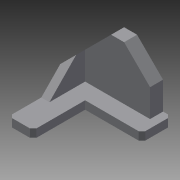
# Autodesk Inventor part: z-axis-bottom
Saved by Autodesk Inventor 2015 (Build 190159000, 159)
## iProperties
Created: 2015-05-29
Part Number: z-axis-bottom
Material: Generic
Document SubType Name: Modeling
Designer: X
Density: 1 g/cm^3
Appearance: Default
Author: X
Autodesk Inventor part; units mm, degrees
ref_plane "YZ Plane" through (0, 0, 0) normal (1, 0, 0) x (0, 1, 0)
ref_plane "XZ Plane" through (0, 0, 0) normal (0, 1, 0) x (-1, 0, 0)
ref_plane "XY Plane" through (0, 0, 0) normal (0, 0, 1) x (1, 0, 0)
sketch "Sketch2" plane through (0, 0, 0) normal (0, 0, 1) x (1, 0, 0)
  line L0 (0, 0) -> (50, 0)
  line L1 (50, 0) -> (50, 50)
  line L2 (50, 50) -> (0, 50)
  line L3 (0, 50) -> (0, 0)
  dimension "d0" = 50
  dimension "d1" = 50
  constraints: 8 end point, 2 parallel, 1 horizontal, 1 perpendicular
  measures "d0" distance of L2.end L0.start
  measures "d1" distance of L0.start L0.end
extrude "Extrusion1" add sketch "Sketch2" along normal blind 38
sketch "Sketch3" plane through (0, 0, 38) normal (0, 0, 1) x (1, 0, 0)
  line L0 (50, 0) -> (15, 0)
  line L1 (15, 0) -> (15, 32)
  line L2 (15, 32) -> (50, 32)
  line L3 (50, 32) -> (50, 0)
  line L4 (0, 50) -> (0, 0) projected
  line L5 (50, 50) -> (0, 50) projected
  dimension "d4" = 15
  dimension "d5" = 18
  constraints: 8 end point, 2 parallel, 1 horizontal, 1 perpendicular
  measures "d4" distance between parallel lines of L4 L1
  measures "d5" distance between parallel lines of L5 L2
extrude "Extrusion2" cut sketch "Sketch3" against normal through all
sketch "Sketch4" plane through (0, 0, 38) normal (0, 0, 1) x (1, 0, 0)
  line L0 (50, 32) -> (50, 50) projected
  line L1 (0, 0) -> (15, 0) projected
  line L2 (50, 42) -> (5, 42)
  line L3 (50, 50) -> (0, 50) projected
  line L4 (5, 42) -> (5, 0)
  line L5 (0, 50) -> (0, 0) projected
  line L6 (5, 0) -> (50, 0)
  line L7 (50, 0) -> (50, 42)
  dimension "d8" = 8
  dimension "d9" = 5
  constraints: 8 end point, 2 horizontal, 2 point on line, 1 perpendicular, 1 vertical
  measures "d8" distance between parallel lines of L2 L3
  measures "d9" distance between parallel lines of L5 L4
extrude "Extrusion3" cut sketch "Sketch4" against normal blind 33 contours L7 L6 L1 L4 L2 L0
sketch "Sketch6" plane through (0, 0, 0) normal (0, 1, 0) x (-1, 0, 0)
  line L0 (0, 17) -> (-21, 38)
  line L1 (-21, 38) -> (-29, 38)
  line L2 (0, 0) -> (0, 38) projected
  line L3 (-29, 38) -> (-45, 22)
  line L4 (-5, 38) -> (-50, 38) projected
  line L5 (-45, 22) -> (-45, 5)
  line L6 (-45, 5) -> (-50, 5)
  line L7 (-50, 5) -> (-50, 0)
  line L8 (-50, 0) -> (0, 0)
  line L9 (0, 17) -> (0, 0)
  dimension "d12" = 8
  dimension "d13" = 5
  dimension "d14" = 5
  dimension "d15" = 135
  dimension "d16" = 135
  dimension "d17" = 17
  constraints: 16 end point, 5 perpendicular, 1 collinear, 1 point on line, 1 vertical
  measures "d12" distance of L0.end L1.end
  measures "d13" distance of L5.end L6.end
  measures "d14" distance of L6.end L7.end
  measures "d15" angle of L5 L3
  measures "d16" angle of L2 L0
  measures "d17" distance of L3.end L5.end
extrude "Extrusion4" cut sketch "Sketch6" along normal through all keep common part
sketch "Sketch8" plane through (0, 0, 0) normal (1, 0, 0) x (0, 1, 0)
  line L0 (42, 38) -> (42, 22)
  line L1 (42, 22) -> (36.5, 22)
  line L2 (36.5, 22) -> (20, 5)
  line L3 (20, 5) -> (0, 5)
  line L4 (0, 5) -> (0, 38)
  line L5 (0, 38) -> (42, 38)
  line L6 (42, 22) -> (42, 38) projected
  line L7 (42, 38) -> (50, 38) projected
  line L8 (0, 22) -> (42, 22) projected
  line L9 (0, 0) -> (0, 17) projected
  dimension "d20" = 17
  dimension "d21" = 5.5
  dimension "d22" = 20
  constraints: 12 end point, 4 collinear, 2 parallel, 2 perpendicular, 1 vertical
  measures "d20" distance between parallel lines of L3 L1
  measures "d21" distance of L0.end L1.end
  measures "d22" distance of L2.end L3.end
extrude "Extrusion5" cut sketch "Sketch8" along normal through all
chamfer "Chamfer1" distance 2 angle 45 1 edges at (0, 0, 2.5)
chamfer "Chamfer2" distance 2 angle 45 1 edges at (15, 0, 2.5)
chamfer "Chamfer3" distance 2 angle 45 1 edges at (50, 32, 2.5)
chamfer "Chamfer4" distance 2 angle 45 1 edges at (50, 50, 2.5)
body "Solid1"
